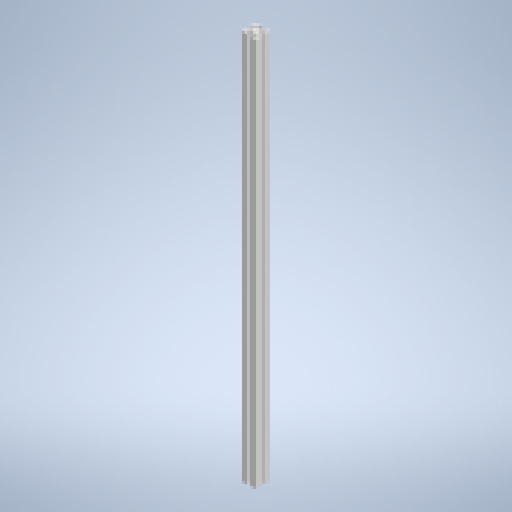
# Autodesk Inventor part: 3030型材
Saved by Autodesk Inventor 2023 (Build 270158000, 158)
## iProperties
Created: 2022-04-16
Part Number: 3030型材
Material: 常规
Document SubType Name: Modeling
Designer: Zhong
Density: 1 g/cm^3
Appearance: 默认
Author: Zhong
Autodesk Inventor part; units mm, degrees
ref_plane "YZ Plane" through (0, 0, 0) normal (1, 0, 0) x (0, 1, 0)
ref_plane "XZ Plane" through (0, 0, 0) normal (0, 1, 0) x (-1, 0, 0)
ref_plane "XY Plane" through (0, 0, 0) normal (0, 0, 1) x (1, 0, 0)
sketch "草图1" plane through (0, 0, 0) normal (0, 1, 0) x (-1, 0, 0)
  line L0 (15, 3.0233) -> (15, 15)
  line L1 (15, 15) -> (3.0233, 15)
  line L2 (3.0233, 15) -> (3.0233, 13.2)
  line L3 (3.0233, 13.2) -> (8.4, 13.2)
  line L4 (8.4, 13.2) -> (8.4, 9.7)
  line L5 (8.4, 9.7) -> (4.4, 5.7)
  line L6 (4.4, 5.7) -> (0, 5.7)
  line L7 (15, 3.0233) -> (13.2, 3.0233)
  line L8 (13.2, 3.0233) -> (13.2, 8.4)
  line L9 (13.2, 8.4) -> (9.7, 8.4)
  line L10 (9.7, 8.4) -> (5.7, 4.4)
  line L11 (5.7, 4.4) -> (5.7, 0)
  line L12 (-15, 3.0233) -> (-13.2, 3.0233)
  line L13 (-5.7, 4.4) -> (-5.7, 0)
  line L14 (-13.2, 3.0233) -> (-13.2, 8.4)
  line L15 (-13.2, 8.4) -> (-9.7, 8.4)
  line L16 (-9.7, 8.4) -> (-5.7, 4.4)
  line L17 (-8.4, 9.7) -> (-4.4, 5.7)
  line L18 (-4.4, 5.7) -> (0, 5.7)
  line L19 (-15, 15) -> (-15, 3.0233)
  line L20 (-8.4, 13.2) -> (-8.4, 9.7)
  line L21 (-3.0233, 15) -> (-15, 15)
  line L22 (-3.0233, 13.2) -> (-8.4, 13.2)
  line L23 (-3.0233, 15) -> (-3.0233, 13.2)
  line L24 (-3.0233, -15) -> (-3.0233, -13.2)
  line L25 (-4.4, -5.7) -> (0, -5.7)
  line L26 (-3.0233, -13.2) -> (-8.4, -13.2)
  line L27 (-8.4, -13.2) -> (-8.4, -9.7)
  line L28 (-8.4, -9.7) -> (-4.4, -5.7)
  line L29 (-9.7, -8.4) -> (-5.7, -4.4)
  line L30 (-5.7, -4.4) -> (-5.7, 0)
  line L31 (-15, -15) -> (-3.0233, -15)
  line L32 (-13.2, -8.4) -> (-9.7, -8.4)
  line L33 (-15, -3.0233) -> (-15, -15)
  line L34 (-13.2, -3.0233) -> (-13.2, -8.4)
  line L35 (-15, -3.0233) -> (-13.2, -3.0233)
  line L36 (15, -3.0233) -> (13.2, -3.0233)
  line L37 (5.7, -4.4) -> (5.7, 0)
  line L38 (13.2, -3.0233) -> (13.2, -8.4)
  line L39 (13.2, -8.4) -> (9.7, -8.4)
  line L40 (9.7, -8.4) -> (5.7, -4.4)
  line L41 (8.4, -9.7) -> (4.4, -5.7)
  line L42 (4.4, -5.7) -> (0, -5.7)
  line L43 (15, -15) -> (15, -3.0233)
  line L44 (8.4, -13.2) -> (8.4, -9.7)
  line L45 (3.0233, -15) -> (15, -15)
  line L46 (3.0233, -13.2) -> (8.4, -13.2)
  line L47 (3.0233, -15) -> (3.0233, -13.2)
  point P0 (0, 0)
  point P1 (15, 0)
  point P2 (0, 0)
  point P3 (0, 0)
  point P4 (0, 0)
  point P5 (0, 0)
  point P6 (0, 0)
  point P7 (0, 15)
  point P8 (0, 0)
  point P9 (0, 0)
  point P10 (0, 0)
  point P11 (-15, 0)
  point P12 (0, 0)
  point P13 (0, 0)
  point P14 (0, 0)
  point P15 (0, -15)
  point P16 (-5.7, 0)
  point P17 (0, -5.7)
  point P18 (5.7, 0)
  dimension "d8" = 5.7
  dimension "d9" = 1.8
  dimension "d10" = 8.4
  dimension "d11" = 4
  dimension "d14" = 360
  constraints: 96 end point, 4 point on line, 2 coincident, 2 perpendicular, 1 parallel, 1 vertical, 115 other
  measures "d8" distance of point (0, 0) L6.end
  measures "d9" distance of L1.end L2.end
  measures "d10" horizontal distance of point (0, 0) L3.end
  measures "d11" horizontal distance of L4.end L5.end
extrude "拉伸1" add sketch "草图1" along normal blind 800
